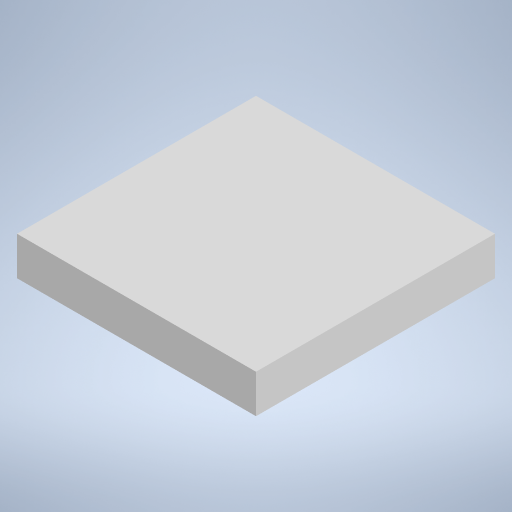
# Autodesk Inventor part: silicon_mold
Saved by Autodesk Inventor 2023.1 (Build 271208000, 208)
## iProperties
Created: 2022-08-08
Part Number: silicon_mold
Material: Generic
Document SubType Name: Modeling
Designer: fraaw
Density: 1 g/cm^3
Appearance: Default
Author: fraaw
## iProperties of the stored document silicon_mold_3DPrint.ipt
Created: 2022-08-08
Part Number: silicon_mold_3DPrint
Material: Generic
Document SubType Name: Modeling
Designer: fraaw
Density: 1 g/cm^3
Appearance: Default
Author: fraaw
Autodesk Inventor part; units mm, degrees
ref_plane "YZ Plane" through (0, 0, 0) normal (1, 0, 0) x (0, 1, 0)
ref_plane "XZ Plane" through (0, 0, 0) normal (0, 1, 0) x (-1, 0, 0)
ref_plane "XY Plane" through (0, 0, 0) normal (0, 0, 1) x (1, 0, 0)
sketch "Sketch1" plane through (0, 0, 0) normal (0, 1, 0) x (-1, 0, 0)
  line L0 (-16.3, 16.3) -> (16.3, 16.3)
  line L1 (16.3, 16.3) -> (16.3, -16.3)
  line L2 (16.3, -16.3) -> (-16.3, -16.3)
  line L3 (-16.3, -16.3) -> (-16.3, 16.3)
  line L4 (-16.3, 16.3) -> (16.3, -16.3) construction
  line L5 (16.3, 16.3) -> (-16.3, -16.3) construction
  line L6 (14.8, 14.8) -> (-14.8, 14.8)
  line L7 (-14.8, 14.8) -> (-14.8, -14.8)
  line L8 (-14.8, -14.8) -> (14.8, -14.8)
  line L9 (14.8, -14.8) -> (14.8, 14.8)
  point P0 (0, 0)
  dimension "d2" = 1.5
  dimension "d31" = 29.6
  dimension "d32" = 29.6
  constraints: 20 end point, 4 parallel, 2 midpoint, 2 perpendicular, 1 horizontal, 3 other
  measures "d2" distance between parallel lines of L0 L6
  measures "d31" distance of L8.end L6.start
  measures "d32" distance of L6.start L6.end
extrude "Extrusion1" add sketch "Sketch1" along normal blind 3.25
sketch "Sketch2" plane through (0, 3.25, 0) normal (0, 1, 0) x (1, 0, 0)
  line L0 (-16.3, 16.3) -> (-16.3, -16.3) projected
  line L1 (-16.3, -16.3) -> (16.3, -16.3) projected
  line L2 (16.3, -16.3) -> (16.3, 16.3) projected
  line L3 (16.3, 16.3) -> (-16.3, 16.3) projected
  point P0 (0, 0)
extrude "Extrusion2" add sketch "Sketch2" along normal blind 2
sketch "Sketch3" plane through (0, 3.25, 0) normal (0, -1, 0) x (1, 0, 0)
  line L0 (-14.8, 14.8) -> (-14.8, -14.8) projected
  line L1 (14.8, 14.8) -> (-14.8, 14.8) projected
  point P0 (0, 0)
  point P1 (-11.85, 11.85)
  point P2 (-8.9, 11.85)
  point P3 (-5.95, 11.85)
  point P4 (-3, 11.85)
  point P5 (-0.05, 11.85)
  point P6 (2.9, 11.85)
  point P7 (5.85, 11.85)
  point P8 (8.8, 11.85)
  point P9 (11.75, 11.85)
  point P10 (-11.85, 8.9)
  point P11 (-8.9, 8.9)
  point P12 (-5.95, 8.9)
  point P13 (-3, 8.9)
  point P14 (-0.05, 8.9)
  point P15 (2.9, 8.9)
  point P16 (5.85, 8.9)
  point P17 (8.8, 8.9)
  point P18 (11.75, 8.9)
  point P19 (-11.85, 5.95)
  point P20 (-8.9, 5.95)
  point P21 (-5.95, 5.95)
  point P22 (-3, 5.95)
  point P23 (-0.05, 5.95)
  point P24 (2.9, 5.95)
  point P25 (5.85, 5.95)
  point P26 (8.8, 5.95)
  point P27 (11.75, 5.95)
  point P28 (-11.85, 3)
  point P29 (-8.9, 3)
  point P30 (-5.95, 3)
  point P31 (-3, 3)
  point P32 (-0.05, 3)
  point P33 (2.9, 3)
  point P34 (5.85, 3)
  point P35 (8.8, 3)
  point P36 (11.75, 3)
  point P37 (-11.85, 0.05)
  point P38 (-8.9, 0.05)
  point P39 (-5.95, 0.05)
  point P40 (-3, 0.05)
  point P41 (-0.05, 0.05)
  point P42 (2.9, 0.05)
  point P43 (5.85, 0.05)
  point P44 (8.8, 0.05)
  point P45 (11.75, 0.05)
  point P46 (-11.85, -2.9)
  point P47 (-8.9, -2.9)
  point P48 (-5.95, -2.9)
  point P49 (-3, -2.9)
  point P50 (-0.05, -2.9)
  point P51 (2.9, -2.9)
  point P52 (5.85, -2.9)
  point P53 (8.8, -2.9)
  point P54 (11.75, -2.9)
  point P55 (-11.85, -5.85)
  point P56 (-8.9, -5.85)
  point P57 (-5.95, -5.85)
  point P58 (-3, -5.85)
  point P59 (-0.05, -5.85)
  point P60 (2.9, -5.85)
  point P61 (5.85, -5.85)
  point P62 (8.8, -5.85)
  point P63 (11.75, -5.85)
  point P64 (-11.85, -8.8)
  point P65 (-8.9, -8.8)
  point P66 (-5.95, -8.8)
  point P67 (-3, -8.8)
  point P68 (-0.05, -8.8)
  point P69 (2.9, -8.8)
  point P70 (5.85, -8.8)
  point P71 (8.8, -8.8)
  point P72 (11.75, -8.8)
  point P73 (-11.85, -11.75)
  point P74 (-8.9, -11.75)
  point P75 (-5.95, -11.75)
  point P76 (-3, -11.75)
  point P77 (-0.05, -11.75)
  point P78 (2.9, -11.75)
  point P79 (5.85, -11.75)
  point P80 (8.8, -11.75)
  point P81 (11.75, -11.75)
  dimension "d7" = 2.95
  dimension "d8" = 2.95
  dimension "d11" = 2.95
  dimension "d14" = 2.95
  constraints: 1 horizontal, 1 vertical, 80 other
  measures "d7" distance from line of L0 point (-11.85, 11.85)
  measures "d8" distance from line of L1 point (-11.85, 11.85)
  measures "d11" distance of point (-11.85, 11.85) point (-8.9, 11.85)
  measures "d14" distance of point (-11.85, 11.85) point (-11.85, 8.9)
hole "Hole1" at (-11.85, 3.25, 11.85) at (-8.9, 3.25, 11.85) at (-5.95, 3.25, 11.85) at (-3, 3.25, 11.85) at (-0.05, 3.25, 11.85) at (2.9, 3.25, 11.85) at (5.85, 3.25, 11.85) at (8.8, 3.25, 11.85) at (11.75, 3.25, 11.85) at (-11.85, 3.25, 8.9) at (-8.9, 3.25, 8.9) at (-5.95, 3.25, 8.9) at (-3, 3.25, 8.9) at (-0.05, 3.25, 8.9) at (2.9, 3.25, 8.9) at (5.85, 3.25, 8.9) at (8.8, 3.25, 8.9) at (11.75, 3.25, 8.9) at (-11.85, 3.25, 5.95) at (-8.9, 3.25, 5.95) at (-5.95, 3.25, 5.95) at (-3, 3.25, 5.95) at (-0.05, 3.25, 5.95) at (2.9, 3.25, 5.95) at (5.85, 3.25, 5.95) at (8.8, 3.25, 5.95) at (11.75, 3.25, 5.95) at (-11.85, 3.25, 3) at (-8.9, 3.25, 3) at (-5.95, 3.25, 3) at (-3, 3.25, 3) at (-0.05, 3.25, 3) at (2.9, 3.25, 3) at (5.85, 3.25, 3) at (8.8, 3.25, 3) at (11.75, 3.25, 3) at (-11.85, 3.25, 0.05) at (-8.9, 3.25, 0.05) at (-5.95, 3.25, 0.05) at (-3, 3.25, 0.05) at (-0.05, 3.25, 0.05) at (2.9, 3.25, 0.05) at (5.85, 3.25, 0.05) at (8.8, 3.25, 0.05) at (11.75, 3.25, 0.05) at (-11.85, 3.25, -2.9) at (-8.9, 3.25, -2.9) at (-5.95, 3.25, -2.9) at (-3, 3.25, -2.9) at (-0.05, 3.25, -2.9) direction (0, 1, 0) diameter 1.5 depth 0.5 and at (2.9, 3.25, -2.9) (5.85, 3.25, -2.9) (8.8, 3.25, -2.9) (11.75, 3.25, -2.9) (-11.85, 3.25, -5.85) (-8.9, 3.25, -5.85) (-5.95, 3.25, -5.85) (-3, 3.25, -5.85) (-0.05, 3.25, -5.85) (2.9, 3.25, -5.85) (5.85, 3.25, -5.85) (8.8, 3.25, -5.85) (11.75, 3.25, -5.85) (-11.85, 3.25, -8.8) (-8.9, 3.25, -8.8) (-5.95, 3.25, -8.8) (-3, 3.25, -8.8) (-0.05, 3.25, -8.8) (2.9, 3.25, -8.8) (5.85, 3.25, -8.8) (8.8, 3.25, -8.8) (11.75, 3.25, -8.8) (-11.85, 3.25, -11.75) (-8.9, 3.25, -11.75) (-5.95, 3.25, -11.75) (-3, 3.25, -11.75) (-0.05, 3.25, -11.75) (2.9, 3.25, -11.75) (5.85, 3.25, -11.75) (8.8, 3.25, -11.75) (11.75, 3.25, -11.75)
fillet "Fillet1" radius 0.5 1 edges at (-11.85, 3.75, 12.6)
pattern_linear "Rectangular Pattern1" count 9 spacing 2.95 along (1, 0, 0) count 9 spacing 2.95 along (0, 0, -1) of "Fillet1"
sketch "Sketch4" plane through (0, 3.25, 0) normal (0, -1, 0) x (1, 0, 0)
  line L0 (14.8, 14.8) -> (-14.8, 14.8) construction
  line L1 (-14.8, -14.8) -> (14.8, -14.8) construction
  line L2 (-14.8, 14.8) -> (14.8, -14.8) construction
  circle A0 centre (-13.3, 13.3) radius 1.5
  circle A1 centre (-13.3, -13.3) radius 1.5
  circle A2 centre (13.3, -13.3) radius 1.5
  circle A3 centre (13.3, 13.3) radius 1.5
  point P0 (0, 0)
  dimension "d33" = 3
  dimension "d36" = 360
  constraints: 4 centre point, 2 end point, 1 point on line, 1 tangent, 9 other
  measures "d33" diameter of A0
extrude "Extrusion3" add sketch "Sketch4" along normal blind 1
equation "\"d32\" = d31"
equation "\"d7\" = d8"
equation "\"d11\" = d8"
equation "\"d14\" = d11"
equation "\"d30\" = d27"
equation "\"d27\" = 2.95"
body "Solid1"
